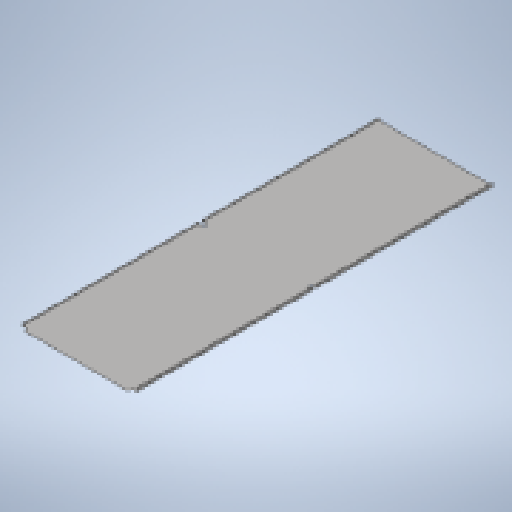
# Autodesk Inventor part: MSC 808 sheet gills
Saved by Autodesk Inventor 2025 (Build 290162010, 162A)
## iProperties
Created: 2024-06-15
Part Number: MSC 808 sheet gills
Material: Stainless Steel
Document SubType Name: Sheet Metal
Designer: pokla
Stock Number: МОО 0101 лист жабра
Mass: 8000 g
Surface Area: 40030 cm^2
Volume: 1000 cm^3
Density: 8 g/cm^3
Sheet Metal Rule: Default_mm
Appearance: Default
Author: pokla
Autodesk Inventor part; units mm, degrees
ref_plane "YZ Plane" through (0, 0, 0) normal (1, 0, 0) x (0, 1, 0)
ref_plane "XZ Plane" through (0, 0, 0) normal (0, 1, 0) x (-1, 0, 0)
ref_plane "XY Plane" through (0, 0, 0) normal (0, 0, 1) x (1, 0, 0)
sketch "Sketch6" plane through (0, 0, 0) normal (0, 1, 0) x (-1, 0, 0)
  line L0 (315, -990) -> (-315, -990)
  line L1 (-315, -990) -> (-315, 990)
  line L2 (-315, 990) -> (315, 990)
  line L3 (315, 990) -> (315, -990)
  line L4 (315, -990) -> (-315, 990) construction
  line L5 (-315, -990) -> (315, 990) construction
  point P0 (0, 0)
  dimension "d52" = 630
  dimension "d53" = 1980
  measures "d52" distance of L1.end L2.end
  measures "d53" distance of L0.end L1.end
extrude "Plate2" add sketch "Sketch6" along normal blind 0.5
sketch "Sketch11" plane through (314.5, 0, -990) normal (1, 0, 0) x (0, 1, 0)
  line L0 (0, 1980) -> (0, 0)
  line L1 (0, 0) -> (10, 0)
  line L2 (10, 0) -> (10, 1980)
  line L3 (10, 1980) -> (0, 1980)
  constraints: 6 end point, 1 horizontal, 1 perpendicular, 1 vertical
edge flange "Flange2" height 10 angle 90 thickness 0.5 bend radius 0.5 thickness toward (1, 0, 0) relief straight relief width 0.5 relief depth 0.25 edges at (315, 0.5, 0) wall of the first edge with corners at (314.5, 0, 990) (314.5, 0, -990) (314.5, 10, -990) (314.5, 10, 990)
bend "Bend3"
corner "Corner3"
sketch "Sketch12" plane through (315, 9.5, -990) normal (0, 1, 0) x (-1, 0, 0)
  line L0 (0, 1980) -> (0, 0)
  line L1 (0, 0) -> (10, 0)
  line L2 (10, 0) -> (10, 1980)
  line L3 (10, 1980) -> (0, 1980)
  constraints: 6 end point, 1 horizontal, 1 perpendicular, 1 vertical
edge flange "Flange3" height 10 angle 90 thickness 0.5 bend radius 0.5 thickness toward (0, 1, 0) relief straight relief width 0.5 relief depth 0.25 edges at (314.5, 10, 0) wall of the first edge with corners at (315, 9.5, 990) (315, 9.5, -990) (305, 9.5, -990) (305, 9.5, 990)
bend "Bend4"
corner "Corner4"
sketch "Sketch13" plane through (-314.5, 0, 990) normal (-1, 0, 0) x (0, -1, 0)
  line L0 (0, -1980) -> (0, 0)
  line L1 (0, 0) -> (-10, 0)
  line L2 (-10, 0) -> (-10, -1980)
  line L3 (-10, -1980) -> (0, -1980)
  constraints: 6 end point, 1 horizontal, 1 perpendicular, 1 vertical
edge flange "Flange4" height 10 angle 90 thickness 0.5 bend radius 0.5 thickness toward (-1, 0, 0) relief straight relief width 0.5 relief depth 0.25 edges at (-315, 0.5, 0) wall of the first edge with corners at (-314.5, 0, -990) (-314.5, 0, 990) (-314.5, 10, 990) (-314.5, 10, -990)
bend "Bend5"
corner "Corner5"
sketch "Sketch14" plane through (-315, 9.5, 990) normal (0, 1, 0) x (-1, 0, 0)
  line L0 (0, -1980) -> (0, 0)
  line L1 (0, 0) -> (-10, 0)
  line L2 (-10, 0) -> (-10, -1980)
  line L3 (-10, -1980) -> (0, -1980)
  constraints: 6 end point, 1 horizontal, 1 perpendicular, 1 vertical
edge flange "Flange5" height 10 angle 90 thickness 0.5 bend radius 0.5 thickness toward (0, 1, 0) relief straight relief width 0.5 relief depth 0.25 edges at (-314.5, 10, 0) wall of the first edge with corners at (-315, 9.5, -990) (-315, 9.5, 990) (-305, 9.5, 990) (-305, 9.5, -990)
bend "Bend6"
corner "Corner6"
sketch "Sketch15" plane through (0, 0, 0) normal (0, -1, 0) x (1, 0, 0)
  line L0 (-315, 990) -> (-285, 990)
  line L1 (-285, 970) -> (-315, 970)
  line L2 (-315, 970) -> (-315, 990)
  line L3 (315, 0) -> (285, 0)
  line L4 (-315, 0) -> (-285, 0)
  line L5 (285, 0) -> (285, -20)
  line L6 (-285, 0) -> (-285, -20)
  line L7 (285, -20) -> (315, -20)
  line L8 (-315, -20) -> (-315, 0)
  line L9 (-285, -20) -> (-315, -20)
  line L10 (315, -20) -> (315, 0)
  line L11 (-285, 990) -> (-285, 970)
  line L12 (285, 970) -> (315, 970)
  line L13 (315, 970) -> (315, 990)
  line L14 (315, 990) -> (285, 990)
  line L15 (285, 990) -> (285, 970)
  line L16 (-314, 990) -> (314, 990) projected
  line L17 (315, 990) -> (315, -990) projected
  line L18 (-315, -990) -> (-315, 990) projected
  point P0 (0, 0)
  dimension "d124" = 20
  dimension "d125" = 30
  dimension "d126" = 990
  dimension "d127" = 30
  constraints: 32 end point, 9 collinear, 8 parallel, 4 horizontal, 4 perpendicular, 3 equal length
  measures "d124" distance of L0.end L1.start
  measures "d125" distance of L0.start L0.end
  measures "d126" distance between parallel lines of L4 L0
  measures "d127" distance of L15.end L12.end
extrude "Extrusion3" cut sketch "Sketch15" against normal through all
fillet "Corner Round1" radius 4 16 edges at (285, 0.25, 990) (285, 0.25, 970) (305, 9.75, 970) (305, 9.75, -20) (285, 0.25, -20) (305, 9.75, 0) (285, 0.25, 0) (305, 9.75, -990) (-305, 9.75, -990) (-305, 9.75, -20) (-285, 0.25, -20) (-285, 0.25, 0) (-305, 9.75, 0) (-305, 9.75, 970) (-285, 0.25, 970) (-285, 0.25, 990)
equation "\"d53\" = ЖАБРЫ_базовая_длина_дл_лист"
equation "\"d127\" = d125"
equation "\"d54\" = Thickness"
equation "\"d84\" = BendReliefWidth"
equation "\"d85\" = BendReliefDepth"
equation "\"d86\" = MinimumRemnant"
equation "\"d87\" = TransitionRadius"
equation "\"d90\" = BendRadius"
equation "\"d91\" = CornerReliefSize"
equation "\"d92\" = GapSize"
equation "\"d93\" = JacobiRadiusSize"
equation "\"d94\" = BendReliefWidth"
equation "\"d95\" = BendReliefDepth"
equation "\"d96\" = MinimumRemnant"
equation "\"d97\" = TransitionRadius"
equation "\"d100\" = BendRadius"
equation "\"d101\" = CornerReliefSize"
equation "\"d102\" = GapSize"
equation "\"d103\" = JacobiRadiusSize"
equation "\"d104\" = BendReliefWidth"
equation "\"d105\" = BendReliefDepth"
equation "\"d106\" = MinimumRemnant"
equation "\"d107\" = TransitionRadius"
equation "\"d110\" = BendRadius"
equation "\"d111\" = CornerReliefSize"
equation "\"d112\" = GapSize"
equation "\"d113\" = JacobiRadiusSize"
equation "\"d114\" = BendReliefWidth"
equation "\"d115\" = BendReliefDepth"
equation "\"d116\" = MinimumRemnant"
equation "\"d117\" = TransitionRadius"
equation "\"d120\" = BendRadius"
equation "\"d121\" = CornerReliefSize"
equation "\"d122\" = GapSize"
equation "\"d123\" = JacobiRadiusSize"
equation "\"BendRadius\" = Thickness"
equation "\"BendReliefWidth\" = Thickness"
equation "\"BendReliefDepth\" = 0.5 * Thickness"
equation "\"CornerReliefSize\" = 4 * Thickness"
equation "\"MinimumRemnant\" = 2 * Thickness"
equation "\"TransitionRadius\" = BendRadius"
equation "\"JacobiRadiusSize\" = BendRadius"
equation "\"GapSize\" = Thickness"
equation "\"ЖАБРЫ_базовая_длина_дл_лист\" = 1980"
equation "\"Thickness\" = 0.5"
body "Solid2"
